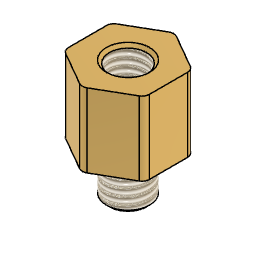
assembly (Autodesk Fusion 360 archive; units mm, degrees)
design "M3 5mm x 3mm standoff"
Autodesk Fusion 360 part; units mm, degrees
sketch "Sketch1" plane through (0, 0, 0) normal (0, 0, 1) x (1, 0, 0)
  circle A0 centre (0, 0) radius 1.5
  line L0 (2.75, 1.5877) -> (0, 3.1754)
  line L1 (0, 3.1754) -> (-2.75, 1.5877)
  line L2 (-2.75, 1.5877) -> (-2.75, -1.5877)
  line L3 (-2.75, -1.5877) -> (0, -3.1754)
  line L4 (0, -3.1754) -> (2.75, -1.5877)
  line L5 (2.75, -1.5877) -> (2.75, 1.5877)
  dimension "d1" = 3
  dimension "d2" = 5.5
  constraint coincident A0.centre origin
  constraint vertical L5
  measures "d1" diameter of A0
  measures "d2" distance of L2 L5
extrude "Extrude1" add sketch "Sketch1" against normal blind 3 contours A0
extrude "Extrude2" add sketch "Sketch1" along normal blind 5 contours A0 | L0 L1 L2 L3 L4 L5
hole "Hole1" at (0, 0, 5) direction (0, 0, -1) diameter 2.529 depth 4 tip angle 118
thread "Thread1" "ISO Metric profile 3.0 M3x0.5 6H"
thread "Thread2" "ISO Metric profile 3.0 M3x0.5 6g" major diameter 2.927 minor diameter 2.3555 pitch 0.5 angle 60 resizes the face on face at (1.4981, -0.0748, -2)
chamfer "Chamfer1" distance 0.2 angle 45 2 edges at (-1.3645, 0.5292, -3) (-1.1789, 0.4573, 5)
fillet "Fillet1" radius 0.5 6 edges at (2.75, -1.5877, 2.5) (2.75, 1.5877, 2.5) (0, -3.1754, 2.5) (0, 3.1754, 2.5) (-2.75, 1.5877, 2.5) (-2.75, -1.5877, 2.5)
